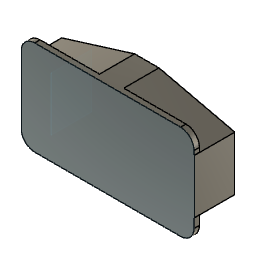
antenna v3 (Autodesk Fusion 360 design; units mm, degrees)
Autodesk Fusion 360 part; units mm, degrees
sketch "Sketch1" plane through (0, 0, 0) normal (0, 1, 0) x (1, 0, 0)
  line L0 (-26, -24) -> (-17, -24)
  line L1 (11.0902, -17.4456) -> (11.0902, 2.573)
  line L2 (-17, 11) -> (-26, 11)
  line L3 (-53, 0.4758) -> (-53, -15.6207)
  line L4 (-53, -15.6207) -> (-26, -24)
  line L5 (-26, 11) -> (-53, 0.4758)
  line L6 (-17, -24) -> (11.0902, -17.4456)
  line L7 (-17, 11) -> (11.0902, 2.573)
  line L8 (-51, -14.5926) -> (-26, -22)
  line L9 (-26, -22) -> (-16.9098, -22)
  line L10 (-16.9098, -22) -> (9.0902, -16.4106)
  line L11 (9.0902, -16.4106) -> (9.0902, 1.5072)
  line L12 (9.0902, 1.5072) -> (-17.1347, 9)
  line L13 (-17.1347, 9) -> (-26.0019, 9)
  line L14 (-26.0019, 9) -> (-51, -0.066)
  line L15 (-51, -0.066) -> (-51, -14.5926)
  dimension "d12" = 2
  dimension "d13" = 2
  dimension "d14" = 2
  dimension "d15" = 2
  dimension "d16" = 25
  dimension "d17" = 26
  constraint horizontal L0
  constraint vertical L1
  constraint horizontal L2
  constraint vertical L3
  constraint horizontal L9
  constraint perpendicular L9 L11
  constraint perpendicular L11 L13
  constraint parallel L11 L15
  measures "d12" distance of L1 L11
  measures "d13" distance of L3 L15
  measures "d14" distance of L2 L13.end
  measures "d15" distance of L0 L9
  measures "d16" horizontal distance of L8.start L8.end
  measures "d17" horizontal distance of L9.end L10.end
extrude "Extrude1" add sketch "Sketch1" along normal blind 15
sketch "Sketch2" plane through (11.0902, 0, 0) normal (1, 0, 0) x (0, 1, 0)
  line L0 (0, 17.4456) -> (0, -2.573)
  line L1 (0, -2.573) -> (15, -2.573)
  line L2 (15, -2.573) -> (15, 17.4456)
  line L3 (15, 17.4456) -> (0, 17.4456)
sketch "Sketch3" plane through (0, 0, 0) normal (0, 1, 0) x (1, 0, 0)
  line L0 (-53, -24) -> (11, -24)
  line L1 (11, -24) -> (11, 11)
  line L2 (11, 11) -> (-53, 11)
  line L3 (-53, 11) -> (-53, -24)
  dimension "d20" = 64
  constraint horizontal L0
  constraint vertical L1
  constraint horizontal L2
  constraint vertical L3
  measures "d20" distance of L0.start L0.end
extrude "Extrude2" add sketch "Sketch3" along normal blind 2
fillet "Fillet1" radius 5 1 edges at (11, 1, 24)
fillet "Fillet2" radius 5 1 edges at (11, 1, -11)
fillet "Fillet3" radius 5 1 edges at (-53, 1, -11)
fillet "Fillet4" radius 5 1 edges at (-53, 1, 24)
sketch "Sketch4" plane through (0, 0, 0) normal (1, 0, 0) x (0, 1, 0)
move_body "Move1" bodies 1 to x (1, 0, 0) y (0, 1, 0) z (0, 0, 1) at (-11, 0, 0)
move_body "Move2" bodies 1 to x (1, 0, 0) y (0, 1, 0) z (0, 0, 1) at (64, 0, 0)
sketch "Sketch5" plane through (0, 0, 0) normal (0, -1, 0) x (1, 0, 0)
  arc A0 (5, 24) -> (0, 19) centre (5, 19) ccw
  line L0 (0, 19) -> (0, -6)
  arc A1 (0, -6) -> (5, -11) centre (5, -6) ccw
  line L1 (5, -11) -> (27, -11)
  line L2 (27, -11) -> (36, -11)
  line L3 (36, -11) -> (59, -11)
  arc A2 (59, -11) -> (64, -6) centre (59, -6) ccw
  line L4 (64, -6) -> (64, -2.6)
  line L5 (64, -2.6) -> (64.0902, -2.573)
  line L6 (64.0902, -2.573) -> (64.0902, 17.4456)
  line L7 (64.0902, 17.4456) -> (64, 17.4667)
  line L8 (64, 17.4667) -> (64, 19)
  arc A3 (64, 19) -> (59, 24) centre (59, 19) ccw
  line L9 (59, 24) -> (5, 24)
sketch "Sketch6" plane through (0, 0, 0) normal (1, 0, 0) x (0, 1, 0)
  line L0 (15, 14) -> (2, 14)
  line L1 (2, 14) -> (2, 1)
  line L2 (2, 1) -> (15, 1)
  line L3 (15, 1) -> (15, 14)
  constraint horizontal L0
  constraint vertical L1
  constraint horizontal L2
  constraint vertical L3
extrude "Extrude3" cut sketch "Sketch6" along normal blind 2
